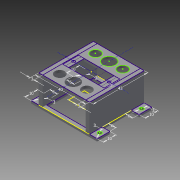
# Autodesk Inventor part: ServoHolder
Saved by Autodesk Inventor 2014 SP1 (Build 180222100, 222)
## iProperties
Created: 2015-03-16
Part Number: ServoHolder
Material: Generic
Document SubType Name: Modeling
Designer: Erin
Density: 1 g/cm^3
Appearance: Default
Author: Erin
Autodesk Inventor part; units mm, degrees
ref_plane "YZ Plane" through (0, 0, 0) normal (1, 0, 0) x (0, 1, 0)
ref_plane "XZ Plane" through (0, 0, 0) normal (0, 1, 0) x (-1, 0, 0)
sketch "Block1_1" plane through (0, 0, 0) normal (0, 0, 1) x (1, 0, 0)
  circle A0 centre (47.029, 24.2723) radius 1.1
  circle A1 centre (75.029, 24.2723) radius 1.1
  line L0 (49.279, 30.4723) -> (72.779, 30.4723)
  line L1 (72.779, 30.4723) -> (72.779, 18.0723)
  line L2 (72.779, 18.0723) -> (49.279, 18.0723)
  line L3 (49.279, 18.0723) -> (49.279, 30.4723)
  line L4 (49.279, 30.4723) -> (44.779, 30.4723)
  line L5 (44.779, 30.4723) -> (44.779, 18.0723)
  line L6 (44.779, 18.0723) -> (49.279, 18.0723)
  line L7 (49.279, 18.0723) -> (49.279, 30.4723)
  line L8 (72.779, 30.4723) -> (77.279, 30.4723)
  line L9 (77.279, 30.4723) -> (77.279, 18.0723)
  line L10 (77.279, 18.0723) -> (72.779, 18.0723)
  line L11 (72.779, 18.0723) -> (72.779, 30.4723)
  line L12 (44.779, 24.2723) -> (77.279, 24.2723) construction
  line L13 (61.029, 30.4723) -> (61.029, 18.0723) construction
  line L14 (47.029, 30.4723) -> (47.029, 18.0723) construction
  line L15 (75.029, 30.4723) -> (75.029, 18.0723) construction
  line L16 (66.779, 30.4723) -> (66.779, 18.0723) construction
  point P0 (60.979, 24.0984)
  dimension "d2" = 23.5
  dimension "d3" = 12.4
  dimension "d4" = 4.5
  dimension "d5" = 4.5
  dimension "d6" = 2.2
  dimension "d7" = 2.2
  dimension "d8" = 2.25
  dimension "d9" = 6
  measures "d2" distance of L1.end L2.end
  measures "d3" distance of L0.end L1.end
  measures "d4" distance of L6.end L5.end
  measures "d5" distance of L9.end L10.end
  measures "d6" diameter of A0
  measures "d7" diameter of A1
  measures "d8" distance between parallel lines of L9 L15
  measures "d9" distance between parallel lines of L16 L1
sketch "Sketch1" plane through (0, 0, 0) normal (0, 0, 1) x (1, 0, 0)
  line L0 (-20, 21.5) -> (20, 21.5)
  line L1 (20, 21.5) -> (20, -21.5)
  line L2 (20, -21.5) -> (-20, -21.5)
  line L3 (-20, -21.5) -> (-20, 21.5)
  line L4 (-0.1493, 33.2365) -> (-0.1493, -35.4112) construction
  line L5 (-27.052, 0) -> (29.4139, 0) construction
  line L6 (20, 21.5) -> (17, 21.5)
  line L7 (17, 21.5) -> (17, -21.5)
  line L8 (17, -21.5) -> (20, -21.5)
  line L9 (20, -21.5) -> (20, 21.5)
  line L10 (-20, 21.5) -> (-17, 21.5)
  line L11 (-17, 21.5) -> (-17, -21.5)
  line L12 (-17, -21.5) -> (-20, -21.5)
  line L13 (-20, -21.5) -> (-20, 21.5)
  line L14 (-20, 21.5) -> (20, 21.5)
  line L15 (20, 21.5) -> (20, -21.5)
  line L16 (20, -21.5) -> (-20, -21.5)
  line L17 (-20, -21.5) -> (-20, 21.5)
  circle A0 centre (-0.1493, 14.0909) radius 4.9337
  circle A1 centre (10.5202, 14.0909) radius 3.8489
  circle A2 centre (-10.8699, 14.0909) radius 3.8489
  circle A3 centre (-14.1493, 0) radius 1.1
  circle A4 centre (13.8507, 0) radius 1.1
  line L18 (-11.8993, 6.2) -> (11.6007, 6.2)
  line L19 (11.6007, 6.2) -> (11.6007, -6.2)
  line L20 (11.6007, -6.2) -> (-11.8993, -6.2)
  line L21 (-11.8993, -6.2) -> (-11.8993, 6.2)
  line L22 (-11.8993, 6.2) -> (-16.3993, 6.2)
  line L23 (-16.3993, 6.2) -> (-16.3993, -6.2)
  line L24 (-16.3993, -6.2) -> (-11.8993, -6.2)
  line L25 (-11.8993, -6.2) -> (-11.8993, 6.2)
  line L26 (11.6007, 6.2) -> (16.1007, 6.2)
  line L27 (16.1007, 6.2) -> (16.1007, -6.2)
  line L28 (16.1007, -6.2) -> (11.6007, -6.2)
  line L29 (11.6007, -6.2) -> (11.6007, 6.2)
  line L30 (-16.3993, 0) -> (16.1007, 0) construction
  line L31 (-0.1493, 6.2) -> (-0.1493, -6.2) construction
  line L32 (-14.1493, 6.2) -> (-14.1493, -6.2) construction
  line L33 (13.8507, 6.2) -> (13.8507, -6.2) construction
  line L34 (5.6007, 6.2) -> (5.6007, -6.2) construction
  point P0 (0, 0)
  point P1 (-20, 0)
  point P2 (0, -21.5)
  dimension "d0" = 40
  dimension "d1" = 43
  dimension "d10" = 3
  dimension "d11" = 3
  constraints: 36 end point, 8 parallel, 6 horizontal, 5 perpendicular, 3 centre point, 3 point on line, 2 midpoint, 2 vertical, 1 horizontal alignment, 1 vertical alignment
  measures "d0" distance of L1.end L2.end
  measures "d1" distance of L0.end L1.end
  measures "d10" distance of L8.end L7.end
  measures "d11" distance of L11.end L12.end
extrude "Extrusion1" add sketch "Sketch1" against normal blind 2 contours L0 L7 L2 L11 | A0 | A1 | A2 | A3 | A4 | L21 L24 L23 L22 | L26 L27 L28 L19
extrude "Extrusion2" add sketch "Sketch1" against normal blind 22 contours L0 L11 L2 L3 | L0 L1 L2 L7
ref_plane "Work Plane1" through (0, 0, -22) normal (0, 0, 1) x (1, 0, 0)
sketch "Sketch2" plane through (0, 0, -22) normal (0, 0, 1) x (1, 0, 0)
  line L0 (-11.8993, 6.2) -> (11.6007, 6.2) projected
  line L1 (11.6007, -6.2) -> (-11.8993, -6.2) projected
  line L2 (20, 21.5) -> (-20, 21.5) projected
  line L3 (-20, 21.5) -> (-20, -21.5) projected
  line L4 (-20, -21.5) -> (20, -21.5) projected
  line L5 (20, -21.5) -> (20, 21.5) projected
  line L6 (-17, 18.5) -> (17, 18.5)
  line L7 (17, 18.5) -> (17, -18.5)
  line L8 (17, -18.5) -> (-17, -18.5)
  line L9 (-17, -18.5) -> (-17, 18.5)
  line L10 (20, 21.5) -> (26, 21.5)
  line L11 (26, 21.5) -> (26, 11.5)
  line L12 (26, 11.5) -> (20, 11.5)
  line L13 (20, 11.5) -> (20, 21.5)
  line L14 (20, -21.5) -> (26, -21.5)
  line L15 (26, -21.5) -> (26, -11.5)
  line L16 (26, -11.5) -> (20, -11.5)
  line L17 (20, -11.5) -> (20, -21.5)
  line L18 (-20, 21.5) -> (-26, 21.5)
  line L19 (-26, 21.5) -> (-26, 11.5)
  line L20 (-26, 11.5) -> (-20, 11.5)
  line L21 (-20, 11.5) -> (-20, 21.5)
  line L22 (-20, -21.5) -> (-26, -21.5)
  line L23 (-26, -21.5) -> (-26, -11.5)
  line L24 (-26, -11.5) -> (-20, -11.5)
  line L25 (-20, -11.5) -> (-20, -21.5)
  circle A0 centre (-23, 16.5) radius 1.5
  circle A1 centre (-23, -16.5) radius 1.5
  circle A2 centre (23, 16.5) radius 1.5
  circle A3 centre (23, -16.5) radius 1.5
  line L26 (-11.8993, -6.2) -> (-11.8993, 6.2) projected
  line L27 (11.6007, 6.2) -> (11.6007, -6.2) projected
  point P0 (0, 0)
  dimension "d17" = 3
  dimension "d22" = 6
  dimension "d23" = 10
  dimension "d24" = 6
  dimension "d25" = 10
  dimension "d26" = 6
  dimension "d27" = 10
  dimension "d28" = 6
  dimension "d29" = 10
  dimension "d30" = 3
  dimension "d31" = 3
  dimension "d32" = 3
  dimension "d33" = 3
  constraints: 40 end point, 8 parallel, 4 centre point, 4 horizontal, 4 perpendicular, 3 other
  measures "d17" distance between parallel lines of L6 L2
  measures "d22" distance of L11.end L12.end
  measures "d23" distance of L10.end L11.end
  measures "d24" distance of L16.end L15.end
  measures "d25" distance of L15.end L14.end
  measures "d26" distance of L20.end L19.end
  measures "d27" distance of L19.end L18.end
  measures "d28" distance of L23.end L24.end
  measures "d29" distance of L22.end L23.end
  measures "d30" diameter of A0
  measures "d31" diameter of A1
  measures "d32" diameter of A2
  measures "d33" diameter of A3
extrude "Extrusion3" add sketch "Sketch2" against normal blind 2 contours L5 L4 L3 L2
extrude "Extrusion4" cut sketch "Sketch1" against normal blind 2 contours A0 | A1 | A2
mirror "Mirror1" about plane through (0, 0, 0) normal (0, 1, 0) of "Extrusion4"
extrude "Extrusion5" add sketch "Sketch2" against normal blind 2 contours L10 L11 L12 L5 | L3 L20 L19 L18 | L16 L15 L14 L5 | L3 L22 L23 L24
body "Solid1"
